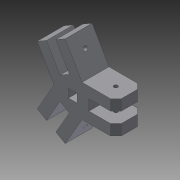
# Autodesk Inventor part: Plunger2
Saved by Autodesk Inventor 2014 SP1 (Build 180222100, 222)
## iProperties
Created: 2014-01-25
Part Number: Plunger2
Material: Generic
Document SubType Name: Modeling
Designer: tom
Density: 1 g/cm^3
Appearance: Default
Author: tom
Autodesk Inventor part; units mm, degrees
ref_plane "YZ Plane" through (0, 0, 0) normal (1, 0, 0) x (0, 1, 0)
ref_plane "XZ Plane" through (0, 0, 0) normal (0, 1, 0) x (-1, 0, 0)
ref_plane "XY Plane" through (0, 0, 0) normal (0, 0, 1) x (1, 0, 0)
sketch "Sketch1" plane through (0, 0, 0) normal (0, 0, 1) x (1, 0, 0)
  line L0 (3.4641, -6) -> (11.0268, -6)
  line L1 (11.0268, -2) -> (6.0268, -2)
  line L2 (6.0268, -2) -> (6.0268, 2)
  line L3 (6.0268, 2) -> (11.0268, 2)
  line L4 (11.0268, 6) -> (3.4641, 6)
  line L5 (16.0268, 2) -> (16.0268, 6)
  line L6 (16.0268, -6) -> (16.0268, -2)
  line L7 (16.0268, 6) -> (3.4641, 6)
  line L8 (3.4641, 6) -> (0, 0)
  line L9 (0, 0) -> (3.4641, -6)
  line L10 (3.4641, -6) -> (16.0268, -6)
  line L11 (16.0268, 2) -> (6.0268, 2)
  line L12 (6.0268, 2) -> (6.0268, -2)
  line L13 (6.0268, -2) -> (16.0268, -2)
  line L14 (16.0268, 6) -> (16.0268, 2)
  line L15 (16.0268, -2) -> (16.0268, -6)
  point P0 (0, 0)
  dimension "d8" = 10
  dimension "d9" = 10
  constraints: 32 end point, 5 perpendicular, 1 parallel
  measures "d8" distance from line of L2.end L5
  measures "d9" distance from line of L1.end L6
extrude "Extrusion1" add sketch "Sketch1" along normal blind 10
chamfer "Chamfer2" distance 2 angle 45 4 edges at (16.0268, 4, 10) (16.0268, -4, 10) (16.0268, -4, 0) (16.0268, 4, 0)
sketch "Sketch3" plane through (3.4641, 6, 10) normal (0, 1, 0) x (1, 0, 0)
  line L0 (10.5627, 10) -> (0, 10) projected
  line L1 (12.5627, 8) -> (12.5627, 2) projected
  circle A0 centre (7.5627, 5) radius 0.75
  point P0 (-3.4641, 10)
  dimension "d13" = 1.5
  dimension "d14" = 5
  dimension "d15" = 5
  constraints: 1 centre point
  measures "d13" diameter of A0
  measures "d14" distance from line of L1 A0.centre
  measures "d15" distance from line of L0 A0.centre
extrude "Extrusion2" cut sketch "Sketch3" against normal blind 22.7
pattern_circular "Circular Pattern1" count 3 over 360 about axis through (0, 0, 0) along (0, 0, 1) of "Extrusion1", "Extrusion2", "Chamfer2"
sketch "Sketch4" plane through (0, 0, 10) normal (0, 0, 1) x (1, 0, 0)
  circle A0 centre (0, 0) radius 0.75
  dimension "d21" = 1.5
  constraints: 1 centre point, 1 coincident
  measures "d21" diameter of A0
extrude "Extrusion3" cut sketch "Sketch4" against normal blind 8
sketch "Sketch6" plane through (0, 0, 0) normal (0, 0, -1) x (-1, 0, 0)
  line L0 (-1.5875, 1.5875) -> (1.5875, 1.5875)
  line L1 (1.5875, 1.5875) -> (1.5875, -1.5875)
  line L2 (1.5875, -1.5875) -> (-1.5875, -1.5875)
  line L3 (-1.5875, -1.5875) -> (-1.5875, 1.5875)
  point P0 (0, 0)
  dimension "d25" = 1.5875
  dimension "d26" = 3.175
  dimension "d27" = 3.175
  dimension "d28" = 1.5875
  constraints: 8 end point, 2 parallel, 1 horizontal, 1 perpendicular
  measures "d25" distance from line of L3 point (0, 0)
  measures "d26" distance of L1.end L2.end
  measures "d27" distance of L0.end L1.end
  measures "d28" distance from line of point (0, 0) L0
extrude "Extrusion4" cut sketch "Sketch6" against normal blind 11.1125
body "Solid1"
